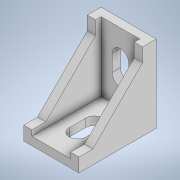
# Autodesk Inventor part: Corner Connector
Saved by Autodesk Inventor 2022 (Build 260153000, 153)
## iProperties
Created: 2021-10-05
Part Number: Corner Connector
Material: Generic
Document SubType Name: Modeling
Designer: Administrator
Density: 1 g/cm^3
Appearance: Default
Mass: 4.34235 g
Surface Area: 34.5474 cm^2
Volume: 4.34235 cm^3
Title: Corner Connector v3
Author: Administrator
Autodesk Inventor part; units mm, degrees
ref_plane "XZ Plane" through (0, 0, 0) normal (0, 1, 0) x (-1, 0, 0)
ref_plane "XY Plane" through (0, 0, 0) normal (0, 0, 1) x (1, 0, 0)
sketch "Sketch1" plane through (0, 0, 0) normal (1, 0, 0) x (0, 1, 0)
  line L0 (28, 5) -> (28, 0)
  line L1 (5, 23) -> (23, 5)
  line L2 (5, 28) -> (5, 23)
  line L3 (0, 0) -> (0, 28)
  line L4 (23, 5) -> (28, 5)
  line L5 (0, 28) -> (5, 28)
  line L6 (28, 0) -> (0, 0)
  constraints: 14 end point, 4 equal length, 3 horizontal, 3 vertical
extrude "Extrusion4" add sketch "Sketch1" along normal blind 20
ref_plane "Work Plane1" through (17, 0, 0) normal (1, 0, 0) x (0, 1, 0)
sketch "Sketch2" plane through (17, 0, 0) normal (1, 0, 0) x (0, 1, 0)
  line L0 (3, 28) -> (3, 3)
  line L1 (5, 23) -> (23, 5)
  line L2 (3, 28) -> (5, 28)
  line L3 (23, 5) -> (28, 5)
  line L4 (3, 3) -> (28, 3)
  line L5 (5, 28) -> (5, 23)
  line L6 (28, 5) -> (28, 3)
  constraints: 14 end point, 3 horizontal, 3 perpendicular, 3 vertical
extrude "Extrusion3" cut sketch "Sketch2" against normal blind 14
sketch "Sketch3" plane through (17, 3, 28) normal (0, 1, 0) x (1, 0, 0)
  arc A0 (-10, 9.5) -> (-4, 9.5) centre (-7, 9.5) ccw
  line L0 (-10, 9.5) -> (-10, 15.5)
  arc A1 (-4, 15.5) -> (-10, 15.5) centre (-7, 15.5) ccw
  line L1 (-4, 15.5) -> (-4, 9.5)
  constraints: 4 end point, 4 point on circle, 2 centre point, 2 vertical, 1 equal radius, 1 parallel
extrude "Extrusion2" cut sketch "Sketch3" against normal blind 3
sketch "Sketch4" plane through (0, 0, 0) normal (0, 0, 1) x (1, 0, 0)
  arc A0 (13, 18.5) -> (7, 18.5) centre (10, 18.5) ccw
  arc A1 (7, 12.5) -> (13, 12.5) centre (10, 12.5) ccw
  line L0 (13, 12.5) -> (13, 18.5)
  line L1 (7, 18.5) -> (7, 12.5)
  constraints: 4 end point, 4 point on circle, 2 centre point, 2 vertical, 1 equal radius, 1 parallel
extrude "Extrusion1" cut sketch "Sketch4" along normal blind 3 draft 0
body "Solid3"
